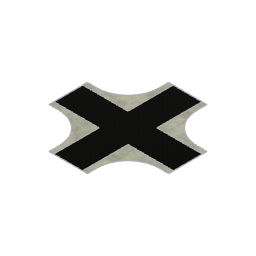
_4 Way.a136dba0-1004-4a8c-b3ed-a23d3a37ed80 (Autodesk Fusion 360 design; units mm, degrees)
Autodesk Fusion 360 part; units mm, degrees
sketch "Sketch1" plane through (0, 0, 0) normal (0, 0, 1) x (1, 0, 0)
  line L0 (406.4, 1270) -> (-406.4, 1270)
  line L1 (-406.4, 1270) -> (-406.4, -1270)
  line L2 (-406.4, -1270) -> (406.4, -1270)
  line L3 (406.4, -1270) -> (406.4, 1270)
  line L4 (406.4, 1270) -> (-406.4, -1270) construction
  line L5 (-406.4, 1270) -> (406.4, -1270) construction
  line L6 (-1270, 406.4) -> (1270, 406.4)
  line L7 (1270, 406.4) -> (1270, -406.4)
  line L8 (1270, -406.4) -> (-1270, -406.4)
  line L9 (-1270, -406.4) -> (-1270, 406.4)
  line L10 (-1270, 406.4) -> (1270, -406.4) construction
  line L11 (1270, 406.4) -> (-1270, -406.4) construction
  line L12 (-1270, 304.8) -> (1270, 304.8)
  line L13 (1270, 304.8) -> (1270, -304.8)
  line L14 (1270, -304.8) -> (-1270, -304.8)
  line L15 (-1270, -304.8) -> (-1270, 304.8)
  line L16 (-1270, 304.8) -> (1270, -304.8) construction
  line L17 (1270, 304.8) -> (-1270, -304.8) construction
  line L18 (304.8, 1270) -> (-304.8, 1270)
  line L19 (-304.8, 1270) -> (-304.8, -1270)
  line L20 (-304.8, -1270) -> (304.8, -1270)
  line L21 (304.8, -1270) -> (304.8, 1270)
  line L22 (304.8, 1270) -> (-304.8, -1270) construction
  line L23 (-304.8, 1270) -> (304.8, -1270) construction
  dimension "d3" = 812.8
  dimension "d4" = 2540
  dimension "d5" = 2540
  dimension "d6" = 609.6
  dimension "d7" = 609.6
  constraint horizontal L0
  constraint perpendicular L0 L1
  constraint parallel L0 L2
  constraint parallel L1 L3
  constraint coincident L4 origin
  constraint coincident L5 origin
  constraint horizontal L6
  constraint perpendicular L6 L7
  constraint parallel L6 L8
  constraint parallel L7 L9
  constraint coincident L10 origin
  constraint coincident L11 origin
  constraint horizontal L12
  constraint perpendicular L12 L13
  constraint parallel L12 L14
  constraint parallel L13 L15
  constraint coincident L16 origin
  constraint coincident L17 origin
  constraint horizontal L18
  constraint perpendicular L18 L19
  constraint parallel L18 L20
  constraint parallel L19 L21
  constraint coincident L22 origin
  constraint coincident L23 origin
  measures "d3" distance of L1.end L2.end
  measures "d4" distance of L0.end L1.end
  measures "d5" distance of L7.end L8.end
  measures "d6" distance of L12.end L13.end
  measures "d7" distance of L19.end L20.end
extrude "Extrude1" add sketch "Sketch1" along normal blind 6.35 contours L0 L6 L18 L19 L21 | L6 L12 L19 L21 | L3 L7 L12 L13 L14 | L3 L12 L14 L21 | L12 L14 L19 L21 | L1 L12 L14 L19 | L8 L14 L19 L21 | L1 L9 L12 L14 L15 | L2 L8 L19 L20 L21
extrude "Extrude2" add sketch "Sketch1" along normal blind 6.096 contours L0 L3 L6 L21 | L3 L6 L7 L12 | L3 L6 L12 L21 | L0 L1 L6 L19 | L1 L6 L12 L19 | L3 L7 L8 L14 | L3 L8 L14 L21 | L1 L6 L9 L12 | L2 L3 L8 L21 | L1 L8 L14 L19 | L1 L8 L9 L14 | L1 L2 L8 L19
fillet "Fillet1" radius 660.4 4 edges at (-406.4, -406.4, 3.048) (406.4, -406.4, 3.048) (406.4, 406.4, 3.048) (-406.4, 406.4, 3.048)
